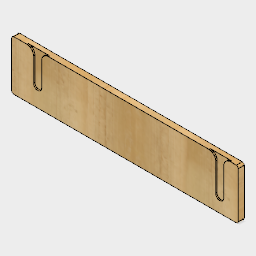
Parallel_Fraesanschlag_2_2_v5 (Autodesk Fusion 360 design; units mm, degrees)
Autodesk Fusion 360 part; units mm, degrees
sketch "Sketch1" plane through (0, 0, 0) normal (0, 0, 1) x (1, 0, 0)
  line L0 (6, 0) -> (674, 0)
  line L1 (680, 6) -> (680, 144)
  line L2 (674, 150) -> (6, 150)
  line L3 (0, 144) -> (0, 6)
  arc A0 (6, 150) -> (0, 144) centre (6, 144) ccw
  arc A1 (680, 144) -> (674, 150) centre (674, 144) ccw
  arc A2 (674, 0) -> (680, 6) centre (674, 6) ccw
  arc A3 (0, 6) -> (6, 0) centre (6, 6) ccw
  point P0 (680, 0)
  point P1 (0, 150)
  dimension "d44" = 680
  dimension "d45" = 150
  dimension "d46" = 6
  measures "d44" distance of origin P0
  measures "d45" distance of origin P1
  measures "d46" radius of A0
extrude "Extrude4" add sketch "Sketch1" along normal blind 14
sketch "pf" plane through (0, 0, 14) normal (0, 0, 1) x (1, 0, 0)
  arc A0 (66, 58) -> (90, 58) centre (78, 58) ccw
  arc A1 (0, 144) -> (6, 150) centre (6, 144) cw
  arc A2 (680, 6) -> (674, 0) centre (674, 6) cw
  line L0 (636, 45) -> (636, 130)
  line L1 (6, 150) -> (46, 150)
  line L2 (656, 150) -> (674, 150)
  line L3 (0, 6) -> (0, 144)
  arc A3 (612, 45) -> (636, 45) centre (624, 45) ccw
  arc A4 (636, 130) -> (656, 150) centre (656, 130) cw
  line L4 (680, 144) -> (680, 6)
  arc A5 (90, 130) -> (110, 150) centre (110, 130) cw
  line L5 (612, 130) -> (612, 45)
  line L6 (110, 150) -> (592, 150)
  arc A6 (592, 150) -> (612, 130) centre (592, 130) cw
  arc A7 (46, 150) -> (66, 130) centre (46, 130) cw
  arc A8 (6, 0) -> (0, 6) centre (6, 6) cw
  arc A9 (674, 150) -> (680, 144) centre (674, 144) cw
  line L7 (674, 0) -> (6, 0)
  line L8 (66, 130) -> (66, 58)
  line L9 (90, 58) -> (90, 130)
extrude "Extrude5" add sketch "pf" along normal blind 4
named bodies: "Body1"
